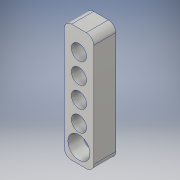
# Autodesk Inventor part: Arm
Saved by Autodesk Inventor 2016 (Build 200138000, 138)
## iProperties
Created: 2015-05-26
Part Number: Arm
Material: Aluminum 6061
Document SubType Name: Modeling
Designer: Jason
Mass: 12.073 g
Surface Area: 28.8868 cm^2
Volume: 4.47149 cm^3
Density: 2.7 g/cm^3
Appearance: Aluminum - Flat
Author: Jason
Autodesk Inventor part; units mm, degrees
ref_plane "YZ Plane" through (0, 0, 0) normal (1, 0, 0) x (0, 1, 0)
ref_plane "XZ Plane" through (0, 0, 0) normal (0, 1, 0) x (-1, 0, 0)
ref_plane "XY Plane" through (0, 0, 0) normal (0, 0, 1) x (1, 0, 0)
sketch "Sketch1" plane through (0, 0, 0) normal (0, 0, 1) x (1, 0, 0)
  line L0 (-6.35, 0) -> (6.35, 0)
  line L1 (6.35, 0) -> (6.35, 50.8)
  line L2 (6.35, 50.8) -> (-6.35, 50.8)
  line L3 (-6.35, 50.8) -> (-6.35, 0)
  point P0 (0, 0)
  dimension "d6" = 50.8
  dimension "d7" = 12.7
  dimension "d22" = 6.35
  constraints: 8 end point, 2 parallel, 1 horizontal, 1 perpendicular
  measures "d6" distance of L0.end L1.end
  measures "d7" distance of L0.start L0.end
  measures "d22" distance of L0.start point (0, 0)
extrude "Stock Bar" add sketch "Sketch1" along normal blind 9.525
sketch "Sketch4" plane through (0, 0, 0) normal (0, 0, -1) x (-1, 0, 0)
  line L0 (6.35, 0) -> (-6.35, 0) projected
  line L1 (-6.35, 0) -> (-6.35, 50.8) projected
  point P0 (0, 0)
  point P1 (0, 6.35)
  dimension "d13" = 6.35
  dimension "d14" = 6.35
  measures "d13" distance from line of L0 point (0, 6.35)
  measures "d14" distance from line of L1 point (0, 6.35)
hole "Motor Hole" at (0, 6.35, 0) direction (0, 0, 1) diameter 6.5278 end through all
sketch "Sketch6" plane through (0, 0, 9.525) normal (0, 0, 1) x (1, 0, 0)
  circle A0 centre (0, 6.35) radius 3.2639 projected
  circle A1 centre (0, 6.35) radius 4.7625
  point P0 (0, 0)
  dimension "d25" = 9.525
  constraints: 1 centre point, 1 coincident
  measures "d25" diameter of A1
extrude "Motor Hole Secondary" cut sketch "Sketch6" against normal blind 6.35
sketch "Sketch5" plane through (0, 0, 9.525) normal (0, 0, 1) x (1, 0, 0)
  line L0 (-6.35, 50.8) -> (-6.35, 0) projected
  line L1 (-6.35, 25.4) -> (6.35, 25.4) construction
  line L2 (6.35, 0) -> (6.35, 50.8) projected
  point P0 (0, 0)
  constraints: 2 end point, 2 midpoint
fillet "Round Edges" radius 3.175 4 edges at (-6.35, 50.8, 4.7625) (6.35, 50.8, 4.7625) (6.35, 0, 4.7625) (-6.35, 0, 4.7625)
pattern_linear "Mounting Holes" count 5 spacing 8.89 along (0, 1, 0) of "Motor Hole"
sketch "Sketch7" plane through (0, 0, 9.525) normal (0, 0, 1) x (1, 0, 0)
  line L0 (-6.35, 47.625) -> (-6.35, 3.175) projected
  line L1 (-6.35, 25.4) -> (6.35, 25.4) construction
  line L2 (6.35, 3.175) -> (6.35, 47.625) projected
  line L3 (0, 25.4) -> (0, 0) construction
  line L4 (-3.175, 0) -> (3.175, 0) projected
  constraints: 4 end point, 3 midpoint, 1 perpendicular
body "Solid2"
